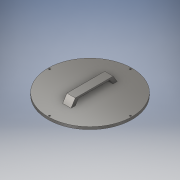
# Autodesk Inventor part: Avi Bay Lid
Saved by Autodesk Inventor 2017 (Build 210142000, 142)
## iProperties
Created: 2016-11-08
Part Number: Avi Bay Lid
Material: Steel, Alloy
Document SubType Name: Modeling
Designer: mnweir
Density: 7.73 g/cm^3
Appearance: Semi-Polished
Author: mnweir
Autodesk Inventor part; units mm, degrees
ref_plane "YZ Plane" through (0, 0, 0) normal (1, 0, 0) x (0, 1, 0)
ref_plane "XZ Plane" through (0, 0, 0) normal (0, 1, 0) x (-1, 0, 0)
sketch "Sketch1" plane through (0, 0, 0) normal (0, 1, 0) x (-1, 0, 0)
  circle A0 centre (0, 0) radius 127
  dimension "d0" = 254
  constraints: 1 centre point, 1 coincident
  measures "d0" diameter of A0
extrude "Extrusion1" add sketch "Sketch1" along normal mid plane 7.62
sketch "Sketch2" plane through (0, 3.81, 0) normal (0, 1, 0) x (1, 0, 0)
  line L0 (0, 0) -> (0, -63.5)
  line L1 (12.7, -69.85) -> (-12.7, -69.85)
  line L2 (-12.7, -69.85) -> (-12.7, -57.15)
  line L3 (-12.7, -57.15) -> (12.7, -57.15)
  line L4 (12.7, -57.15) -> (12.7, -69.85)
  line L5 (12.7, -69.85) -> (-12.7, -57.15) construction
  line L6 (-12.7, -69.85) -> (12.7, -57.15) construction
  dimension "d4" = 63.5
  dimension "d5" = 12.7
  dimension "d6" = 25.4
  constraints: 14 end point, 2 midpoint, 2 parallel, 1 horizontal, 1 perpendicular, 1 vertical
  measures "d4" distance of L0.start L0.end
  measures "d5" distance of L1.end L2.end
  measures "d6" distance of L1.start L1.end
ref_plane "Work Plane1" through (0, 24.13, 0) normal (0, 1, 0) x (1, 0, 0)
sketch "Sketch3" plane through (0, 24.13, 0) normal (0, 1, 0) x (1, 0, 0)
  line L0 (0, 0) -> (0, -50.8)
  line L1 (12.7, -57.15) -> (-12.7, -57.15)
  line L2 (-12.7, -57.15) -> (-12.7, -44.45)
  line L3 (-12.7, -44.45) -> (12.7, -44.45)
  line L4 (12.7, -44.45) -> (12.7, -57.15)
  line L5 (12.7, -57.15) -> (-12.7, -44.45) construction
  line L6 (-12.7, -57.15) -> (12.7, -44.45) construction
  dimension "d8" = 50.8
  dimension "d9" = 12.7
  dimension "d10" = 25.4
  constraints: 14 end point, 2 midpoint, 2 parallel, 1 horizontal, 1 perpendicular, 1 vertical
  measures "d8" distance of L0.start L0.end
  measures "d9" distance of L1.end L2.end
  measures "d10" distance of L1.start L1.end
loft "Loft1" add profiles "Sketch2", "Sketch3"
sketch "Sketch4" plane through (0, 0, 0) normal (0, 0, 1) x (1, 0, 0)
  line L0 (0, 0) -> (0, 24.13)
  line L1 (12.7, 24.13) -> (-12.7, 24.13) projected
  line L2 (0, 24.13) -> (0, 21.59)
  line L3 (-12.7, 19.05) -> (12.7, 19.05)
  line L4 (12.7, 19.05) -> (12.7, 24.13)
  line L5 (12.7, 24.13) -> (-12.7, 24.13)
  line L6 (-12.7, 24.13) -> (-12.7, 19.05)
  line L7 (-12.7, 19.05) -> (12.7, 24.13) construction
  line L8 (12.7, 19.05) -> (-12.7, 24.13) construction
  dimension "d15" = 2.54
  dimension "d16" = 25.4
  constraints: 16 end point, 3 midpoint, 2 parallel, 2 point on line, 1 horizontal, 1 perpendicular
  measures "d15" distance of L0.end L2.end
  measures "d16" distance of L3.start L3.end
extrude "Extrusion2" add sketch "Sketch4" along normal up to next
mirror "Mirror1" about plane through (0, 0, 0) normal (0, 0, 1) of "Loft1", "Extrusion2"
sketch "Sketch5" plane through (0, 3.81, 0) normal (0, 1, 0) x (1, 0, 0)
  line L0 (0, 0) -> (-122.1674, 0)
  dimension "d19" = 122.1674
  constraints: 2 end point, 1 horizontal
  measures "d19" distance of L0.start L0.end
hole "Hole1" at (-122.1674, 3.81, 0) direction (0, -1, 0) diameter 4.9784 depth 19.05 tip angle 118 thread size "1/4-20 UNC" class "2B" standard "ANSI Unified Screw Threads"
pattern_circular "Circular Pattern1" count 4 over 360 about axis through (0, -10, 0) along (0, 1, 0) of "Hole1"
body "Solid1"
